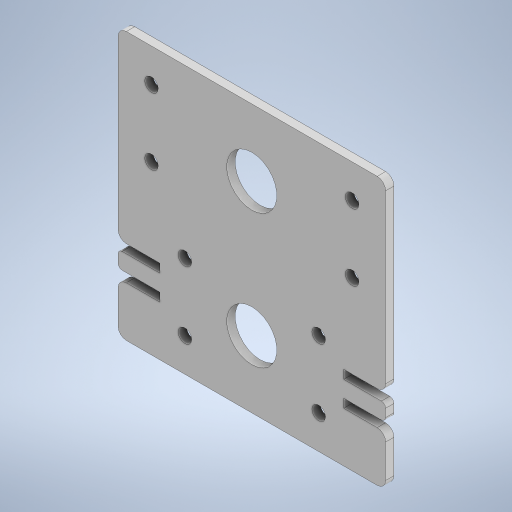
# Autodesk Inventor part: Dipper Plate (backplate)
Saved by Autodesk Inventor 2023 (Build 270158000, 158)
## iProperties
Created: 2023-03-02
Part Number: Dipper Plate (backplate)
Material: Generic
Document SubType Name: Modeling
Designer: Gabriel - T3 CAD
Density: 1 g/cm^3
Appearance: Default
Author: Gabriel - T3 CAD
Autodesk Inventor part; units mm, degrees
ref_plane "YZ Plane" through (0, 0, 0) normal (1, 0, 0) x (0, 1, 0)
ref_plane "XZ Plane" through (0, 0, 0) normal (0, 1, 0) x (-1, 0, 0)
ref_plane "XY Plane" through (0, 0, 0) normal (0, 0, 1) x (1, 0, 0)
sketch "Sketch2" plane through (0, 0, 0) normal (0, 0, 1) x (1, 0, 0)
  line L0 (0, 0) -> (-101.6, 0)
  line L1 (-101.6, 0) -> (-101.6, 101.6)
  line L2 (-101.6, 101.6) -> (0, 101.6)
  line L3 (0, 101.6) -> (0, 0)
  circle A0 centre (-12.7, 88.9) radius 2.5797
  circle A1 centre (-50.8, 76.2) radius 9.525
  circle A2 centre (-25.4, 38.1) radius 2.5797
  circle A3 centre (-50.8, 25.4) radius 9.525
  circle A4 centre (-88.9, 88.9) radius 2.5797
  circle A5 centre (-12.7, 63.5) radius 2.5797
  circle A6 centre (-88.9, 63.5) radius 2.5797
  circle A7 centre (-76.2, 38.1) radius 2.5797
  circle A8 centre (-25.4, 12.7) radius 2.5797
  circle A9 centre (-76.2, 12.7) radius 2.5797
  line L4 (-85.725, 19.05) -> (-101.6, 19.05)
  line L5 (-101.6, 19.05) -> (-101.6, 22.225)
  line L6 (-101.6, 22.225) -> (-85.725, 22.225)
  line L7 (-85.725, 22.225) -> (-85.725, 19.05)
  line L8 (-101.6, 22.225) -> (-85.725, 22.225)
  line L9 (-85.725, 22.225) -> (-85.725, 23.8125)
  line L10 (-85.725, 23.8125) -> (-101.6, 23.8125)
  line L11 (-101.6, 23.8125) -> (-101.6, 22.225)
  line L12 (-85.725, 23.8125) -> (-101.6, 23.8125)
  line L13 (-101.6, 23.8125) -> (-101.6, 26.9875)
  line L14 (-101.6, 26.9875) -> (-85.725, 26.9875)
  line L15 (-85.725, 26.9875) -> (-85.725, 23.8125)
  line L16 (-101.6, 26.9875) -> (-85.725, 26.9875)
  line L17 (-85.725, 26.9875) -> (-85.725, 28.575)
  line L18 (-85.725, 28.575) -> (-101.6, 28.575)
  line L19 (-101.6, 28.575) -> (-101.6, 26.9875)
  line L20 (-85.725, 28.575) -> (-101.6, 28.575)
  line L21 (-101.6, 28.575) -> (-101.6, 31.75)
  line L22 (-101.6, 31.75) -> (-85.725, 31.75)
  line L23 (-85.725, 31.75) -> (-85.725, 28.575)
  line L24 (-85.725, 31.8135) -> (-101.6, 31.8135)
  line L25 (-101.6, 31.8135) -> (-101.6, 28.5115)
  line L26 (-101.6, 28.5115) -> (-85.725, 28.5115)
  line L27 (-85.725, 28.5115) -> (-85.725, 31.8135)
  line L28 (-85.725, 27.051) -> (-101.6, 27.051)
  line L29 (-101.6, 27.051) -> (-101.6, 23.749)
  line L30 (-101.6, 23.749) -> (-85.725, 23.749)
  line L31 (-85.725, 23.749) -> (-85.725, 27.051)
  line L32 (-85.725, 22.2885) -> (-101.6, 22.2885)
  line L33 (-101.6, 22.2885) -> (-101.6, 18.9865)
  line L34 (-101.6, 18.9865) -> (-85.725, 18.9865)
  line L35 (-85.725, 18.9865) -> (-85.725, 22.2885)
  line L36 (-101.6, 26.4583) -> (-85.725, 26.4583)
  line L37 (-85.725, 26.4583) -> (-85.725, 24.3417)
  line L38 (-85.725, 24.3417) -> (-101.6, 24.3417)
  line L39 (-101.6, 24.3417) -> (-101.6, 26.4583)
  line L40 (-50.8, 0) -> (-50.8, 101.6)
  line L41 (-15.875, 19.05) -> (0, 19.05)
  line L42 (0, 19.05) -> (0, 22.225)
  line L43 (0, 22.225) -> (-15.875, 22.225)
  line L44 (-15.875, 22.225) -> (-15.875, 19.05)
  line L45 (0, 22.225) -> (-15.875, 22.225)
  line L46 (-15.875, 22.225) -> (-15.875, 23.8125)
  line L47 (-15.875, 23.8125) -> (0, 23.8125)
  line L48 (0, 23.8125) -> (0, 22.225)
  line L49 (-15.875, 23.8125) -> (0, 23.8125)
  line L50 (0, 23.8125) -> (0, 26.9875)
  line L51 (0, 26.9875) -> (-15.875, 26.9875)
  line L52 (-15.875, 26.9875) -> (-15.875, 23.8125)
  line L53 (0, 26.9875) -> (-15.875, 26.9875)
  line L54 (-15.875, 26.9875) -> (-15.875, 28.575)
  line L55 (-15.875, 28.575) -> (0, 28.575)
  line L56 (0, 28.575) -> (0, 26.9875)
  line L57 (-15.875, 28.575) -> (0, 28.575)
  line L58 (0, 28.575) -> (0, 31.75)
  line L59 (0, 31.75) -> (-15.875, 31.75)
  line L60 (-15.875, 31.75) -> (-15.875, 28.575)
  line L61 (-15.875, 31.8135) -> (0, 31.8135)
  line L62 (0, 31.8135) -> (0, 28.5115)
  line L63 (0, 28.5115) -> (-15.875, 28.5115)
  line L64 (-15.875, 28.5115) -> (-15.875, 31.8135)
  line L65 (-15.875, 27.051) -> (0, 27.051)
  line L66 (0, 27.051) -> (0, 23.749)
  line L67 (0, 23.749) -> (-15.875, 23.749)
  line L68 (-15.875, 23.749) -> (-15.875, 27.051)
  line L69 (-15.875, 22.2885) -> (0, 22.2885)
  line L70 (0, 22.2885) -> (0, 18.9865)
  line L71 (0, 18.9865) -> (-15.875, 18.9865)
  line L72 (-15.875, 18.9865) -> (-15.875, 22.2885)
  line L73 (0, 26.4583) -> (-15.875, 26.4583)
  line L74 (-15.875, 26.4583) -> (-15.875, 24.3417)
  line L75 (-15.875, 24.3417) -> (0, 24.3417)
  line L76 (0, 24.3417) -> (0, 26.4583)
  point P0 (-101.6, 30.1625)
  point P1 (-101.6, 20.6375)
  point P2 (-101.6, 25.4)
  point P3 (-85.725, 25.4)
  point P4 (0, 30.1625)
  point P5 (0, 20.6375)
  point P6 (0, 25.4)
  point P7 (-15.875, 25.4)
  point P8 (-50.8, 15.875)
  point P9 (-50.8, 34.925)
  point P10 (-50.8, 66.675)
  point P11 (-50.8, 85.725)
  dimension "d60" = 101.6
  dimension "d61" = 101.6
  dimension "d62" = 19.05
  dimension "d63" = 5.1594
  dimension "d66" = 12.7
  dimension "d69" = 76.2
  dimension "d72" = 25.4
  dimension "d75" = 12.7
  dimension "d76" = 38.1
  dimension "d77" = 12.7
  dimension "d80" = 50.8
  dimension "d83" = 25.4
  dimension "d86" = 25.4
  dimension "d87" = 12.7
  dimension "d88" = 12.7
  dimension "d89" = 25.4
  dimension "d96" = 3.175
  dimension "d97" = 1.5875
  dimension "d98" = 3.302
  dimension "d101" = 2.1167
  dimension "d103" = 15.875
  dimension "d104" = 25.4
  constraints: 154 end point, 40 symmetric about line, 20 parallel, 12 horizontal, 11 equal length, 10 centre point, 10 midpoint, 10 perpendicular, 10 point on line, 6 collinear, 2 equal radius, 2 vertical, 12 other
  measures "d60" distance of L1.end L2.end
  measures "d61" distance of L0.end L1.end
  measures "d62" diameter of A1
  measures "d63" diameter of A0
  measures "d66" distance from line of L3 A0.centre
  measures "d69" distance of A0.centre A4.centre
  measures "d72" distance of A0.centre A5.centre
  measures "d75" distance from line of L2 A0.centre
  measures "d76" horizontal distance of A0.centre A1.centre
  measures "d77" vertical distance of A0.centre A1.centre
  measures "d80" distance of A2.centre A7.centre
  measures "d83" distance of A2.centre A8.centre
  measures "d86" distance from line of L3 A2.centre
  measures "d87" distance from line of L0 A8.centre
  measures "d88" vertical distance of A8.centre A3.centre
  measures "d89" horizontal distance of A8.centre A3.centre
  measures "d96" distance of L6.end L4.start
  measures "d97" distance of L10.end L8.start
  measures "d98" distance of L34.end L32.start
  measures "d101" distance of L36.end L37.end
  measures "d103" distance of L25.end L26.end
  measures "d104" distance from line of L0 point (-85.725, 25.4)
extrude "Extrusion2" add sketch "Sketch2" along normal blind 3.175 contours L0 L40 A3 A1 L2 L3 L61 L64 L60 L54 L52 L46 L44 L72 L71 | L0 L1 L34 L35 L7 L9 L15 L17 L23 L27 L24 L2 L40 A1 A3 | L69 L46 L67 L3 | L67 L46 L47 L3 | L1 L30 L9 L32 | L47 L52 L75 L3 | L1 L10 L9 L30 | L75 L52 L73 L3 | L1 L38 L15 L10 | L73 L52 L51 L3 | L1 L36 L15 L38 | L51 L54 L65 L3 | L1 L14 L15 L36 | L65 L54 L63 L3 | L1 L28 L17 L14 | L26 L17 L28 L1
fillet "Fillet3" radius 3.175 8 edges at (0, 101.6, 1.5875) (-101.6, 101.6, 1.5875) (0, 18.9865, 1.5875) (0, 31.8135, 1.5875) (0, 0, 1.5875) (-101.6, 0, 1.5875) (-101.6, 18.9865, 1.5875) (-101.6, 31.8135, 1.5875)
fillet "Fillet4" radius 1.5875 4 edges at (0, 22.2885, 1.5875) (0, 28.5115, 1.5875) (-101.6, 22.2885, 1.5875) (-101.6, 28.5115, 1.5875)
body "Solid2"
